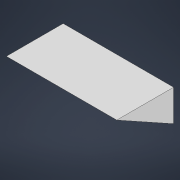
# Autodesk Inventor part: Banco
Saved by Autodesk Inventor 2022 (Build 260153000, 153)
## iProperties
Created: 2022-06-10
Part Number: Banco
Material: Generic
Document SubType Name: Modeling
Designer: Gugarauj07
Density: 1 g/cm^3
Appearance: Default
Author: Gugarauj07
Autodesk Inventor part; units mm, degrees
ref_plane "YZ Plane" through (0, 0, 0) normal (1, 0, 0) x (0, 1, 0)
ref_plane "XZ Plane" through (0, 0, 0) normal (0, 1, 0) x (-1, 0, 0)
ref_plane "XY Plane" through (0, 0, 0) normal (0, 0, 1) x (1, 0, 0)
sketch "Sketch1" plane through (0, 0, 0) normal (0, 0, 1) x (1, 0, 0)
  line L0 (-175, -50) -> (175, -50)
  line L1 (175, -50) -> (175, 50)
  line L2 (175, 50) -> (-175, 50)
  line L3 (-175, 50) -> (-175, -50)
  line L4 (-175, -50) -> (175, 50) construction
  line L5 (175, -50) -> (-175, 50) construction
  point P0 (0, 0)
  dimension "d0" = 350
  dimension "d1" = 100
  constraints: 12 end point, 2 midpoint, 2 parallel, 1 horizontal, 1 perpendicular
  measures "d0" distance of L2.end L1.end
  measures "d1" distance of L1.end L0.end
extrude "Extrusion1" add sketch "Sketch1" along normal blind 180
sketch "Sketch2" plane through (-175, -50, 0) normal (-1, 0, 0) x (0, 0, 1)
  line L0 (180, 0) -> (180, 100) projected
  line L1 (180, 100) -> (0, 0)
  line L2 (0, 0) -> (196.9773, -61.362)
  line L3 (196.9773, -61.362) -> (180, 100)
  point P0 (0, 50)
  constraints: 6 end point
extrude "Extrusion2" cut sketch "Sketch2" against normal through all
body "Solid1"
